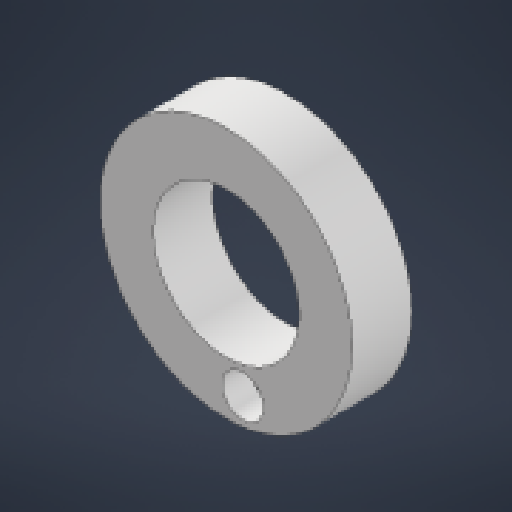
# Autodesk Inventor part: counterbore side
Saved by Autodesk Inventor 2023.2 (Build 272271030, 271C)
## iProperties
Created: 2023-04-05
Part Number: counterbore side
Material: Generic
Document SubType Name: Modeling
Designer: ralph
Density: 1 g/cm^3
Appearance: Default
Author: ralph
Autodesk Inventor part; units mm, degrees
ref_plane "YZ Plane" through (0, 0, 0) normal (1, 0, 0) x (0, 1, 0)
ref_plane "XZ Plane" through (0, 0, 0) normal (0, 1, 0) x (-1, 0, 0)
sketch "Sketch1" plane through (0, 0, 0) normal (0, 0, 1) x (1, 0, 0)
  circle A0 centre (0, -5) radius 24.13
  arc A1 (8.8745, 26.3158) -> (5.7516, 27.0368) centre (0, -5) ccw projected
  arc A2 (4.2323, 24.7681) -> (5.7516, 27.0368) centre (-4.1491, 32.0239) ccw projected
  arc A3 (-2.4071, 24.9709) -> (4.2323, 24.7681) centre (0.994, 27.5338) ccw projected
  arc A4 (-3.7851, 27.3282) -> (-2.4071, 24.9709) centre (6.4016, 31.7016) ccw projected
  arc A5 (-3.7851, 27.3282) -> (-6.9462, 26.7992) centre (0, -5) ccw projected
  arc A6 (-7.4816, 24.1217) -> (-6.9462, 26.7992) centre (-18.0017, 27.6179) ccw projected
  arc A7 (-13.6933, 21.7684) -> (-7.4816, 24.1217) centre (-11.5318, 25.4377) ccw projected
  arc A8 (-15.8684, 23.4189) -> (-13.6933, 21.7684) centre (-8.1308, 31.3576) ccw projected
  arc A9 (-15.8684, 23.4189) -> (-18.5865, 21.7204) centre (0, -5) ccw projected
  arc A10 (-18.0565, 19.0419) -> (-18.5865, 21.7204) centre (-29.1137, 18.246) ccw projected
  arc A11 (-22.8947, 14.4906) -> (-18.0565, 19.0419) centre (-22.302, 18.7078) ccw projected
  arc A12 (-25.5359, 15.183) -> (-22.8947, 14.4906) centre (-21.4253, 25.4785) ccw projected
  arc A13 (-25.5359, 15.183) -> (-27.3971, 12.5737) centre (0, -5) ccw projected
  arc A14 (-25.8825, 10.3019) -> (-27.3971, 12.5737) centre (-35.7934, 5.3352) ccw projected
  arc A15 (-28.6107, 4.2455) -> (-25.8825, 10.3019) centre (-29.677, 8.3685) ccw projected
  arc A16 (-31.3158, 3.8745) -> (-28.6107, 4.2455) centre (-31.4581, 14.9594) ccw projected
  arc A17 (-31.3158, 3.8745) -> (-32.0368, 0.7516) centre (0, -5) ccw projected
  arc A18 (-29.7681, -0.7677) -> (-32.0368, 0.7516) centre (-37.0239, -9.1491) ccw projected
  arc A19 (-29.9709, -7.4071) -> (-29.7681, -0.7677) centre (-32.5338, -4.006) ccw projected
  arc A20 (-32.3282, -8.7851) -> (-29.9709, -7.4071) centre (-36.7016, 1.4016) ccw projected
  arc A21 (-32.3282, -8.7851) -> (-31.7992, -11.9462) centre (0, -5) ccw projected
  arc A22 (-29.1217, -12.4816) -> (-31.7992, -11.9462) centre (-32.6179, -23.0017) ccw projected
  arc A23 (-26.7684, -18.6933) -> (-29.1217, -12.4816) centre (-30.4377, -16.5318) ccw projected
  arc A24 (-28.4189, -20.8684) -> (-26.7684, -18.6933) centre (-36.3576, -13.1308) ccw projected
  arc A25 (-28.4189, -20.8684) -> (-26.7204, -23.5865) centre (0, -5) ccw projected
  arc A26 (-24.0419, -23.0565) -> (-26.7204, -23.5865) centre (-23.246, -34.1137) ccw projected
  arc A27 (-19.4906, -27.8947) -> (-24.0419, -23.0565) centre (-23.7078, -27.302) ccw projected
  arc A28 (-20.183, -30.5359) -> (-19.4906, -27.8947) centre (-30.4785, -26.4253) ccw projected
  arc A29 (-20.183, -30.5359) -> (-17.5737, -32.3971) centre (0, -5) ccw projected
  arc A30 (-15.3019, -30.8825) -> (-17.5737, -32.3971) centre (-10.3352, -40.7934) ccw projected
  arc A31 (-9.2455, -33.6107) -> (-15.3019, -30.8825) centre (-13.3685, -34.677) ccw projected
  arc A32 (-8.8745, -36.3158) -> (-9.2455, -33.6107) centre (-19.9594, -36.4581) ccw projected
  arc A33 (-8.8745, -36.3158) -> (-5.7516, -37.0368) centre (0, -5) ccw projected
  arc A34 (-4.2323, -34.7681) -> (-5.7516, -37.0368) centre (4.1491, -42.0239) ccw projected
  arc A35 (2.4071, -34.9709) -> (-4.2323, -34.7681) centre (-0.994, -37.5338) ccw projected
  arc A36 (3.7851, -37.3282) -> (2.4071, -34.9709) centre (-6.4016, -41.7016) ccw projected
  arc A37 (3.7851, -37.3282) -> (6.9462, -36.7992) centre (0, -5) ccw projected
  arc A38 (7.4816, -34.1217) -> (6.9462, -36.7992) centre (18.0017, -37.6179) ccw projected
  arc A39 (13.6933, -31.7684) -> (7.4816, -34.1217) centre (11.5318, -35.4377) ccw projected
  arc A40 (15.8684, -33.4189) -> (13.6933, -31.7684) centre (8.1308, -41.3576) ccw projected
  arc A41 (15.8684, -33.4189) -> (18.5865, -31.7204) centre (0, -5) ccw projected
  arc A42 (18.0565, -29.0419) -> (18.5865, -31.7204) centre (29.1137, -28.246) ccw projected
  arc A43 (22.8947, -24.4906) -> (18.0565, -29.0419) centre (22.302, -28.7078) ccw projected
  arc A44 (25.5359, -25.183) -> (22.8947, -24.4906) centre (21.4253, -35.4785) ccw projected
  arc A45 (25.5359, -25.183) -> (27.3971, -22.5737) centre (0, -5) ccw projected
  arc A46 (25.8825, -20.3019) -> (27.3971, -22.5737) centre (35.7934, -15.3352) ccw projected
  arc A47 (28.6107, -14.2455) -> (25.8825, -20.3019) centre (29.677, -18.3685) ccw projected
  arc A48 (31.3158, -13.8745) -> (28.6107, -14.2455) centre (31.4581, -24.9594) ccw projected
  arc A49 (31.3158, -13.8745) -> (32.0368, -10.7516) centre (0, -5) ccw projected
  arc A50 (29.7681, -9.2323) -> (32.0368, -10.7516) centre (37.0239, -0.8509) ccw projected
  arc A51 (29.9709, -2.5929) -> (29.7681, -9.2323) centre (32.5338, -5.994) ccw projected
  arc A52 (32.3282, -1.2149) -> (29.9709, -2.5929) centre (36.7016, -11.4016) ccw projected
  arc A53 (32.3282, -1.2149) -> (31.7992, 1.9462) centre (0, -5) ccw projected
  arc A54 (29.1217, 2.4816) -> (31.7992, 1.9462) centre (32.6179, 13.0017) ccw projected
  arc A55 (26.7684, 8.6933) -> (29.1217, 2.4816) centre (30.4377, 6.5318) ccw projected
  arc A56 (28.4189, 10.8684) -> (26.7684, 8.6933) centre (36.3576, 3.1308) ccw projected
  arc A57 (28.4189, 10.8684) -> (26.7204, 13.5865) centre (0, -5) ccw projected
  arc A58 (24.0419, 13.0565) -> (26.7204, 13.5865) centre (23.246, 24.1137) ccw projected
  arc A59 (19.4906, 17.8947) -> (24.0419, 13.0565) centre (23.7078, 17.302) ccw projected
  arc A60 (20.183, 20.5359) -> (19.4906, 17.8947) centre (30.4785, 16.4253) ccw projected
  arc A61 (20.183, 20.5359) -> (17.5737, 22.3971) centre (0, -5) ccw projected
  arc A62 (15.3019, 20.8825) -> (17.5737, 22.3971) centre (10.3352, 30.7934) ccw projected
  arc A63 (9.2455, 23.6107) -> (15.3019, 20.8825) centre (13.3685, 24.677) ccw projected
  arc A64 (8.8745, 26.3158) -> (9.2455, 23.6107) centre (19.9594, 26.4581) ccw projected
  circle A65 centre (0, -5) radius 13.97 projected
  circle A66 centre (-3.1442, 13.7887) radius 2.3813 projected
  circle A67 centre (18.7887, -1.8558) radius 2.3813 projected
  circle A68 centre (-18.7887, -8.1442) radius 2.3813 projected
  circle A69 centre (3.1442, -23.7887) radius 2.3813 projected
  point P0 (0, 0)
  dimension "d0" = 48.26
  constraints: 1 centre point
  measures "d0" diameter of A0
extrude "Extrusion1" add sketch "Sketch1" along normal blind 9.525 contours A0 | A65 | A66 | A67 | A68 | A69
sketch "Sketch2" plane through (0, -5, 9.525) normal (0, 0, 1) x (1, 0, 0)
  circle A0 centre (0, 0) radius 24.13 projected
  circle A1 centre (0, 19.05) radius 4.7625
  circle A2 centre (-19.05, 0) radius 1.27 projected
  circle A3 centre (-19.05, 0) radius 4.7625
  circle A4 centre (19.05, 0) radius 4.7625
  circle A5 centre (0, -19.05) radius 4.7625
  point P0 (0, 5)
  dimension "d3" = 9.525
  dimension "d4" = 9.525
  dimension "d5" = 9.525
  dimension "d6" = 9.525
  constraints: 4 centre point, 1 coincident
  measures "d3" diameter of A1
  measures "d4" diameter of A3
  measures "d5" diameter of A4
  measures "d6" diameter of A5
ref_plane "Work Plane1" through (-23.0187, -8.9687, 4.5858) normal (0, 0, -1) x (0, 1, 0)
extrude "Extrusion2" [suppressed]
sketch "Sketch3" plane through (0, -5, 9.525) normal (0, 0, 1) x (1, 0, 0)
  circle A0 centre (0, 0) radius 13.97
  point P0 (0, 5)
  dimension "d9" = 27.94
  constraints: 1 centre point
  measures "d9" diameter of A0
extrude "Extrusion3" cut sketch "Sketch3" against normal blind 39.6875
sketch "Sketch4" plane through (0, -5, 9.525) normal (0, 0, 1) x (1, 0, 0)
  circle A0 centre (0, 0) radius 13.97 projected
  circle A1 centre (0, 0) radius 24.13 projected
  point P0 (0, 5)
extrude "Extrusion4" add sketch "Sketch4" against normal blind 11.43
sketch "Sketch5" plane through (0, -5, 9.525) normal (0, 0, 1) x (1, 0, 0)
  circle A0 centre (-3.1442, 18.7887) radius 2.3813 projected
  circle A1 centre (18.7887, 3.1442) radius 2.3813 projected
  circle A2 centre (-18.7887, -3.1442) radius 2.3813 projected
  circle A3 centre (3.1442, -18.7887) radius 2.3813 projected
  circle A4 centre (0, 0) radius 13.97 projected
  arc A5 (8.8745, 31.3158) -> (5.7516, 32.0368) centre (0, 0) ccw projected
  arc A6 (4.2323, 29.7681) -> (5.7516, 32.0368) centre (-4.1491, 37.0239) ccw projected
  arc A7 (-2.4071, 29.9709) -> (4.2323, 29.7681) centre (0.994, 32.5338) ccw projected
  arc A8 (-3.7851, 32.3282) -> (-2.4071, 29.9709) centre (6.4016, 36.7016) ccw projected
  arc A9 (-3.7851, 32.3282) -> (-6.9462, 31.7992) centre (0, 0) ccw projected
  arc A10 (-7.4816, 29.1217) -> (-6.9462, 31.7992) centre (-18.0017, 32.6179) ccw projected
  arc A11 (-13.6933, 26.7684) -> (-7.4816, 29.1217) centre (-11.5318, 30.4377) ccw projected
  arc A12 (-15.8684, 28.4189) -> (-13.6933, 26.7684) centre (-8.1308, 36.3576) ccw projected
  arc A13 (-15.8684, 28.4189) -> (-18.5865, 26.7204) centre (0, 0) ccw projected
  arc A14 (-18.0565, 24.0419) -> (-18.5865, 26.7204) centre (-29.1137, 23.246) ccw projected
  arc A15 (-22.8947, 19.4906) -> (-18.0565, 24.0419) centre (-22.302, 23.7078) ccw projected
  arc A16 (-25.5359, 20.183) -> (-22.8947, 19.4906) centre (-21.4253, 30.4785) ccw projected
  arc A17 (-25.5359, 20.183) -> (-27.3971, 17.5737) centre (0, 0) ccw projected
  arc A18 (-25.8825, 15.3019) -> (-27.3971, 17.5737) centre (-35.7934, 10.3352) ccw projected
  arc A19 (-28.6107, 9.2455) -> (-25.8825, 15.3019) centre (-29.677, 13.3685) ccw projected
  arc A20 (-31.3158, 8.8745) -> (-28.6107, 9.2455) centre (-31.4581, 19.9594) ccw projected
  arc A21 (-31.3158, 8.8745) -> (-32.0368, 5.7516) centre (0, 0) ccw projected
  arc A22 (-29.7681, 4.2323) -> (-32.0368, 5.7516) centre (-37.0239, -4.1491) ccw projected
  arc A23 (-29.9709, -2.4071) -> (-29.7681, 4.2323) centre (-32.5338, 0.994) ccw projected
  arc A24 (-32.3282, -3.7851) -> (-29.9709, -2.4071) centre (-36.7016, 6.4016) ccw projected
  arc A25 (-32.3282, -3.7851) -> (-31.7992, -6.9462) centre (0, 0) ccw projected
  arc A26 (-29.1217, -7.4816) -> (-31.7992, -6.9462) centre (-32.6179, -18.0017) ccw projected
  arc A27 (-26.7684, -13.6933) -> (-29.1217, -7.4816) centre (-30.4377, -11.5318) ccw projected
  arc A28 (-28.4189, -15.8684) -> (-26.7684, -13.6933) centre (-36.3576, -8.1308) ccw projected
  arc A29 (-28.4189, -15.8684) -> (-26.7204, -18.5865) centre (0, 0) ccw projected
  arc A30 (-24.0419, -18.0565) -> (-26.7204, -18.5865) centre (-23.246, -29.1137) ccw projected
  arc A31 (-19.4906, -22.8947) -> (-24.0419, -18.0565) centre (-23.7078, -22.302) ccw projected
  arc A32 (-20.183, -25.5359) -> (-19.4906, -22.8947) centre (-30.4785, -21.4253) ccw projected
  arc A33 (-20.183, -25.5359) -> (-17.5737, -27.3971) centre (0, 0) ccw projected
  arc A34 (-15.3019, -25.8825) -> (-17.5737, -27.3971) centre (-10.3352, -35.7934) ccw projected
  arc A35 (-9.2455, -28.6107) -> (-15.3019, -25.8825) centre (-13.3685, -29.677) ccw projected
  arc A36 (-8.8745, -31.3158) -> (-9.2455, -28.6107) centre (-19.9594, -31.4581) ccw projected
  arc A37 (-8.8745, -31.3158) -> (-5.7516, -32.0368) centre (0, 0) ccw projected
  arc A38 (-4.2323, -29.7681) -> (-5.7516, -32.0368) centre (4.1491, -37.0239) ccw projected
  arc A39 (2.4071, -29.9709) -> (-4.2323, -29.7681) centre (-0.994, -32.5338) ccw projected
  arc A40 (3.7851, -32.3282) -> (2.4071, -29.9709) centre (-6.4016, -36.7016) ccw projected
  arc A41 (3.7851, -32.3282) -> (6.9462, -31.7992) centre (0, 0) ccw projected
  arc A42 (7.4816, -29.1217) -> (6.9462, -31.7992) centre (18.0017, -32.6179) ccw projected
  arc A43 (13.6933, -26.7684) -> (7.4816, -29.1217) centre (11.5318, -30.4377) ccw projected
  arc A44 (15.8684, -28.4189) -> (13.6933, -26.7684) centre (8.1308, -36.3576) ccw projected
  arc A45 (15.8684, -28.4189) -> (18.5865, -26.7204) centre (0, 0) ccw projected
  arc A46 (18.0565, -24.0419) -> (18.5865, -26.7204) centre (29.1137, -23.246) ccw projected
  arc A47 (22.8947, -19.4906) -> (18.0565, -24.0419) centre (22.302, -23.7078) ccw projected
  arc A48 (25.5359, -20.183) -> (22.8947, -19.4906) centre (21.4253, -30.4785) ccw projected
  arc A49 (25.5359, -20.183) -> (27.3971, -17.5737) centre (0, 0) ccw projected
  arc A50 (25.8825, -15.3019) -> (27.3971, -17.5737) centre (35.7934, -10.3352) ccw projected
  arc A51 (28.6107, -9.2455) -> (25.8825, -15.3019) centre (29.677, -13.3685) ccw projected
  arc A52 (31.3158, -8.8745) -> (28.6107, -9.2455) centre (31.4581, -19.9594) ccw projected
  arc A53 (31.3158, -8.8745) -> (32.0368, -5.7516) centre (0, 0) ccw projected
  arc A54 (29.7681, -4.2323) -> (32.0368, -5.7516) centre (37.0239, 4.1491) ccw projected
  arc A55 (29.9709, 2.4071) -> (29.7681, -4.2323) centre (32.5338, -0.994) ccw projected
  arc A56 (32.3282, 3.7851) -> (29.9709, 2.4071) centre (36.7016, -6.4016) ccw projected
  arc A57 (32.3282, 3.7851) -> (31.7992, 6.9462) centre (0, 0) ccw projected
  arc A58 (29.1217, 7.4816) -> (31.7992, 6.9462) centre (32.6179, 18.0017) ccw projected
  arc A59 (26.7684, 13.6933) -> (29.1217, 7.4816) centre (30.4377, 11.5318) ccw projected
  arc A60 (28.4189, 15.8684) -> (26.7684, 13.6933) centre (36.3576, 8.1308) ccw projected
  arc A61 (28.4189, 15.8684) -> (26.7204, 18.5865) centre (0, 0) ccw projected
  arc A62 (24.0419, 18.0565) -> (26.7204, 18.5865) centre (23.246, 29.1137) ccw projected
  arc A63 (19.4906, 22.8947) -> (24.0419, 18.0565) centre (23.7078, 22.302) ccw projected
  arc A64 (20.183, 25.5359) -> (19.4906, 22.8947) centre (30.4785, 21.4253) ccw projected
  arc A65 (20.183, 25.5359) -> (17.5737, 27.3971) centre (0, 0) ccw projected
  arc A66 (15.3019, 25.8825) -> (17.5737, 27.3971) centre (10.3352, 35.7934) ccw projected
  arc A67 (9.2455, 28.6107) -> (15.3019, 25.8825) centre (13.3685, 29.677) ccw projected
  arc A68 (8.8745, 31.3158) -> (9.2455, 28.6107) centre (19.9594, 31.4581) ccw projected
  circle A69 centre (3.1442, -18.7887) radius 4.3656
  circle A70 centre (-18.7887, -3.1442) radius 4.3656
  circle A71 centre (18.7887, 3.1442) radius 4.3656
  circle A72 centre (-3.1442, 18.7887) radius 4.3656
  point P0 (0, 5)
  dimension "d14" = 8.7312
  dimension "d17" = 8.7312
  dimension "d18" = 8.7312
  dimension "d19" = 8.7312
  constraints: 4 centre point, 4 coincident
  measures "d14" diameter of A69
  measures "d17" diameter of A70
  measures "d18" diameter of A71
  measures "d19" diameter of A72
extrude "Extrusion5" cut sketch "Sketch5" against normal blind 6.731 contours A0 | A1 | A2 | A3 | A69 | A70 | A71 | A72
sketch "Sketch6" plane through (0, -5, 9.525) normal (0, 0, 1) x (1, 0, 0)
  circle A0 centre (0, 0) radius 24.13 projected
  circle A1 centre (-3.1442, 18.7887) radius 2.3813 projected
  circle A2 centre (18.7887, 3.1442) radius 2.3813 projected
  circle A3 centre (-18.7887, -3.1442) radius 2.3813 projected
  circle A4 centre (3.1442, -18.7887) radius 2.3813 projected
  circle A5 centre (0, 0) radius 13.97 projected
  arc A6 (8.8745, 31.3158) -> (5.7516, 32.0368) centre (0, 0) ccw projected
  arc A7 (4.2323, 29.7681) -> (5.7516, 32.0368) centre (-4.1491, 37.0239) ccw projected
  arc A8 (-2.4071, 29.9709) -> (4.2323, 29.7681) centre (0.994, 32.5338) ccw projected
  arc A9 (-3.7851, 32.3282) -> (-2.4071, 29.9709) centre (6.4016, 36.7016) ccw projected
  arc A10 (-3.7851, 32.3282) -> (-6.9462, 31.7992) centre (0, 0) ccw projected
  arc A11 (-7.4816, 29.1217) -> (-6.9462, 31.7992) centre (-18.0017, 32.6179) ccw projected
  arc A12 (-13.6933, 26.7684) -> (-7.4816, 29.1217) centre (-11.5318, 30.4377) ccw projected
  arc A13 (-15.8684, 28.4189) -> (-13.6933, 26.7684) centre (-8.1308, 36.3576) ccw projected
  arc A14 (-15.8684, 28.4189) -> (-18.5865, 26.7204) centre (0, 0) ccw projected
  arc A15 (-18.0565, 24.0419) -> (-18.5865, 26.7204) centre (-29.1137, 23.246) ccw projected
  arc A16 (-22.8947, 19.4906) -> (-18.0565, 24.0419) centre (-22.302, 23.7078) ccw projected
  arc A17 (-25.5359, 20.183) -> (-22.8947, 19.4906) centre (-21.4253, 30.4785) ccw projected
  arc A18 (-25.5359, 20.183) -> (-27.3971, 17.5737) centre (0, 0) ccw projected
  arc A19 (-25.8825, 15.3019) -> (-27.3971, 17.5737) centre (-35.7934, 10.3352) ccw projected
  arc A20 (-28.6107, 9.2455) -> (-25.8825, 15.3019) centre (-29.677, 13.3685) ccw projected
  arc A21 (-31.3158, 8.8745) -> (-28.6107, 9.2455) centre (-31.4581, 19.9594) ccw projected
  arc A22 (-31.3158, 8.8745) -> (-32.0368, 5.7516) centre (0, 0) ccw projected
  arc A23 (-29.7681, 4.2323) -> (-32.0368, 5.7516) centre (-37.0239, -4.1491) ccw projected
  arc A24 (-29.9709, -2.4071) -> (-29.7681, 4.2323) centre (-32.5338, 0.994) ccw projected
  arc A25 (-32.3282, -3.7851) -> (-29.9709, -2.4071) centre (-36.7016, 6.4016) ccw projected
  arc A26 (-32.3282, -3.7851) -> (-31.7992, -6.9462) centre (0, 0) ccw projected
  arc A27 (-29.1217, -7.4816) -> (-31.7992, -6.9462) centre (-32.6179, -18.0017) ccw projected
  arc A28 (-26.7684, -13.6933) -> (-29.1217, -7.4816) centre (-30.4377, -11.5318) ccw projected
  arc A29 (-28.4189, -15.8684) -> (-26.7684, -13.6933) centre (-36.3576, -8.1308) ccw projected
  arc A30 (-28.4189, -15.8684) -> (-26.7204, -18.5865) centre (0, 0) ccw projected
  arc A31 (-24.0419, -18.0565) -> (-26.7204, -18.5865) centre (-23.246, -29.1137) ccw projected
  arc A32 (-19.4906, -22.8947) -> (-24.0419, -18.0565) centre (-23.7078, -22.302) ccw projected
  arc A33 (-20.183, -25.5359) -> (-19.4906, -22.8947) centre (-30.4785, -21.4253) ccw projected
  arc A34 (-20.183, -25.5359) -> (-17.5737, -27.3971) centre (0, 0) ccw projected
  arc A35 (-15.3019, -25.8825) -> (-17.5737, -27.3971) centre (-10.3352, -35.7934) ccw projected
  arc A36 (-9.2455, -28.6107) -> (-15.3019, -25.8825) centre (-13.3685, -29.677) ccw projected
  arc A37 (-8.8745, -31.3158) -> (-9.2455, -28.6107) centre (-19.9594, -31.4581) ccw projected
  arc A38 (-8.8745, -31.3158) -> (-5.7516, -32.0368) centre (0, 0) ccw projected
  arc A39 (-4.2323, -29.7681) -> (-5.7516, -32.0368) centre (4.1491, -37.0239) ccw projected
  arc A40 (2.4071, -29.9709) -> (-4.2323, -29.7681) centre (-0.994, -32.5338) ccw projected
  arc A41 (3.7851, -32.3282) -> (2.4071, -29.9709) centre (-6.4016, -36.7016) ccw projected
  arc A42 (3.7851, -32.3282) -> (6.9462, -31.7992) centre (0, 0) ccw projected
  arc A43 (7.4816, -29.1217) -> (6.9462, -31.7992) centre (18.0017, -32.6179) ccw projected
  arc A44 (13.6933, -26.7684) -> (7.4816, -29.1217) centre (11.5318, -30.4377) ccw projected
  arc A45 (15.8684, -28.4189) -> (13.6933, -26.7684) centre (8.1308, -36.3576) ccw projected
  arc A46 (15.8684, -28.4189) -> (18.5865, -26.7204) centre (0, 0) ccw projected
  arc A47 (18.0565, -24.0419) -> (18.5865, -26.7204) centre (29.1137, -23.246) ccw projected
  arc A48 (22.8947, -19.4906) -> (18.0565, -24.0419) centre (22.302, -23.7078) ccw projected
  arc A49 (25.5359, -20.183) -> (22.8947, -19.4906) centre (21.4253, -30.4785) ccw projected
  arc A50 (25.5359, -20.183) -> (27.3971, -17.5737) centre (0, 0) ccw projected
  arc A51 (25.8825, -15.3019) -> (27.3971, -17.5737) centre (35.7934, -10.3352) ccw projected
  arc A52 (28.6107, -9.2455) -> (25.8825, -15.3019) centre (29.677, -13.3685) ccw projected
  arc A53 (31.3158, -8.8745) -> (28.6107, -9.2455) centre (31.4581, -19.9594) ccw projected
  arc A54 (31.3158, -8.8745) -> (32.0368, -5.7516) centre (0, 0) ccw projected
  arc A55 (29.7681, -4.2323) -> (32.0368, -5.7516) centre (37.0239, 4.1491) ccw projected
  arc A56 (29.9709, 2.4071) -> (29.7681, -4.2323) centre (32.5338, -0.994) ccw projected
  arc A57 (32.3282, 3.7851) -> (29.9709, 2.4071) centre (36.7016, -6.4016) ccw projected
  arc A58 (32.3282, 3.7851) -> (31.7992, 6.9462) centre (0, 0) ccw projected
  arc A59 (29.1217, 7.4816) -> (31.7992, 6.9462) centre (32.6179, 18.0017) ccw projected
  arc A60 (26.7684, 13.6933) -> (29.1217, 7.4816) centre (30.4377, 11.5318) ccw projected
  arc A61 (28.4189, 15.8684) -> (26.7684, 13.6933) centre (36.3576, 8.1308) ccw projected
  arc A62 (28.4189, 15.8684) -> (26.7204, 18.5865) centre (0, 0) ccw projected
  arc A63 (24.0419, 18.0565) -> (26.7204, 18.5865) centre (23.246, 29.1137) ccw projected
  arc A64 (19.4906, 22.8947) -> (24.0419, 18.0565) centre (23.7078, 22.302) ccw projected
  arc A65 (20.183, 25.5359) -> (19.4906, 22.8947) centre (30.4785, 21.4253) ccw projected
  arc A66 (20.183, 25.5359) -> (17.5737, 27.3971) centre (0, 0) ccw projected
  arc A67 (15.3019, 25.8825) -> (17.5737, 27.3971) centre (10.3352, 35.7934) ccw projected
  arc A68 (9.2455, 28.6107) -> (15.3019, 25.8825) centre (13.3685, 29.677) ccw projected
  arc A69 (8.8745, 31.3158) -> (9.2455, 28.6107) centre (19.9594, 31.4581) ccw projected
  point P0 (0, 5)
extrude "Extrusion6" cut sketch "Sketch6" against normal blind 11.43 contours A1 | A2 | A3 | A4
body "Solid1"
